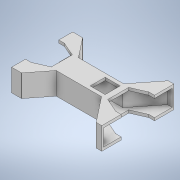
# Autodesk Inventor part: Metal_Shroud
Saved by Autodesk Inventor 2022 (Build 260153000, 153)
## iProperties
Created: 2022-01-23
Part Number: Metal_Shroud
Material: Generic
Document SubType Name: Modeling
Designer: Mlees
Density: 1 g/cm^3
Appearance: Default
Author: Mlees
Autodesk Inventor part; units mm, degrees
ref_plane "YZ Plane" through (0, 0, 0) normal (1, 0, 0) x (0, 1, 0)
ref_plane "XZ Plane" through (0, 0, 0) normal (0, 1, 0) x (-1, 0, 0)
ref_plane "XY Plane" through (0, 0, 0) normal (0, 0, 1) x (1, 0, 0)
sketch "Sketch1" plane through (0, 0, 0) normal (0, 1, 0) x (-1, 0, 0)
  line L0 (172.412, 0) -> (172.412, -65)
  line L1 (172.412, 0) -> (172.412, 65)
  line L2 (172.412, 65) -> (162.412, 65)
  line L3 (162.412, 65) -> (127.012, 20)
  line L4 (172.412, -65) -> (162.412, -65)
  line L5 (162.412, -65) -> (127.012, -20)
  line L6 (127.012, -20) -> (86.206, -20)
  line L7 (127.012, 20) -> (86.206, 20)
  line L8 (0, 0) -> (0, -65)
  line L9 (0, 0) -> (0, 65)
  line L10 (0, 65) -> (10, 65)
  line L11 (10, 65) -> (45.4, 20)
  line L12 (0, -65) -> (10, -65)
  line L13 (10, -65) -> (45.4, -20)
  line L14 (45.4, -20) -> (86.206, -20)
  line L15 (45.4, 20) -> (86.206, 20)
  dimension "d0" = 172.412
  dimension "d1" = 65
  dimension "d2" = 65
  dimension "d7" = 10
  constraints: 32 end point, 2 horizontal, 2 vertical
  measures "d0" distance of point (0, 0) L0.start
  measures "d1" distance of L0.start L0.end
  measures "d2" distance of L0.start L1.end
  measures "d7" distance of L1.end L2.end
extrude "Extrusion1" add sketch "Sketch1" along normal blind 5
sketch "Sketch2" plane through (0, 5, 0) normal (0, 1, 0) x (1, 0, 0)
  line L0 (-162.412, -65) -> (-127.012, -20) projected
  line L1 (-127.012, -20) -> (-162.412, -65)
  line L2 (-162.412, -65) -> (-172.412, -65)
  line L3 (-127.012, 20) -> (-162.412, 65) projected
  line L4 (-172.412, 65) -> (-162.412, 65)
  line L5 (-162.412, 65) -> (-127.012, 20)
  line L6 (-127.012, 20) -> (-45.4, 20)
  line L7 (-10, 65) -> (-45.4, 20) projected
  line L8 (-45.4, 20) -> (-10, 65)
  line L9 (-10, 65) -> (0, 65)
  line L10 (0, -65) -> (0, 65) projected
  line L11 (-45.4, -20) -> (-10, -65) projected
  line L12 (0, -65) -> (-10, -65)
  line L13 (-10, -65) -> (-45.4, -20)
  line L14 (-45.4, -20) -> (-127.012, -20)
  line L15 (-128.469, -17) -> (-163.869, -62)
  line L16 (-163.869, -62) -> (-169.412, -62)
  line L17 (-169.412, 62) -> (-163.869, 62)
  line L18 (-163.869, 62) -> (-128.469, 17)
  line L19 (-128.469, 17) -> (-43.943, 17)
  line L20 (-43.943, 17) -> (-8.543, 62)
  line L21 (-8.543, 62) -> (-3, 62)
  line L22 (-3, -62) -> (-8.543, -62)
  line L23 (-8.543, -62) -> (-43.943, -17)
  line L24 (-43.943, -17) -> (-128.469, -17)
  line L25 (-3, -62) -> (0, -62)
  line L26 (0, -65) -> (0, -62)
  line L27 (-3, 62) -> (0, 62)
  line L28 (0, 65) -> (0, 62)
  line L29 (-169.412, -62) -> (-172.412, -62)
  line L30 (-172.412, -65) -> (-172.412, -62)
  line L31 (-169.412, 62) -> (-172.412, 62)
  line L32 (-172.412, 62) -> (-172.412, 65)
  point P0 (0, 0)
  dimension "d10" = 3
  constraints: 56 end point, 6 parallel, 4 collinear, 3 perpendicular, 1 point on line, 1 vertical, 7 other
  measures "d10" distance between parallel lines of L14 L24
extrude "Extrusion2" add sketch "Sketch2" along normal blind 30
sketch "Sketch3" plane through (0, 35, 0) normal (0, 1, 0) x (1, 0, 0)
  line L0 (-172.412, 65) -> (-172.412, -65) projected
  line L1 (-172.412, -65) -> (-172.412, 65)
  line L2 (-162.412, 65) -> (-172.412, 65) projected
  line L3 (-172.412, 65) -> (-162.412, 65)
  line L4 (-45.4, 20) -> (-127.012, 20) projected
  line L5 (-162.412, 65) -> (-127.012, 20)
  line L6 (-127.012, 20) -> (-45.4, 20)
  line L7 (-45.4, 20) -> (-10, 65)
  line L8 (0, 65) -> (-10, 65) projected
  line L9 (-10, 65) -> (0, 65)
  line L10 (-10, -65) -> (0, -65) projected
  line L11 (0, 65) -> (0, -65)
  line L12 (0, -65) -> (-10, -65)
  line L13 (-127.012, -20) -> (-45.4, -20) projected
  line L14 (-10, -65) -> (-45.4, -20)
  line L15 (-45.4, -20) -> (-127.012, -20)
  line L16 (-162.412, -65) -> (-127.012, -20) projected
  line L17 (-127.012, -20) -> (-162.412, -65)
  line L18 (-172.412, -65) -> (-162.412, -65) projected
  line L19 (-162.412, -65) -> (-172.412, -65)
  point P0 (0, 0)
  constraints: 24 end point, 6 collinear, 2 parallel, 1 perpendicular, 1 vertical
extrude "Extrusion3" add sketch "Sketch3" along normal blind 5
sketch "Sketch4" plane through (0, 40, 0) normal (0, 1, 0) x (1, 0, 0)
  line L0 (0, 0) -> (0, -30)
  line L1 (0, -62) -> (0, 62) projected
  line L2 (0, 0) -> (0, 30)
  line L3 (0, 30) -> (-10, 30)
  line L4 (-35.4, 0) -> (-35.4, 18.85)
  line L5 (-35.4, 18.85) -> (-10, 30)
  line L6 (-35.4, 0) -> (-35.4, -18.85)
  line L7 (-35.4, -18.85) -> (-10, -30)
  line L8 (-10, -30) -> (0, -30)
  line L9 (-127.012, -20) -> (-45.4, -20) projected
  line L10 (-45.4, 20) -> (-127.012, 20) projected
  line L11 (-172.412, 0) -> (-172.412, -30)
  line L12 (-172.412, 0) -> (-172.412, 30)
  line L13 (-172.412, 30) -> (-162.412, 30)
  line L14 (-137.012, 0) -> (-137.012, 18.85)
  line L15 (-137.012, 18.85) -> (-162.412, 30)
  line L16 (-137.012, 0) -> (-137.012, -18.85)
  line L17 (-137.012, -18.85) -> (-162.412, -30)
  line L18 (-162.412, -30) -> (-172.412, -30)
  dimension "d15" = 30
  dimension "d16" = 30
  dimension "d17" = 10
  dimension "d18" = 35.4
  dimension "d19" = 18.85
  dimension "d20" = 18.85
  constraints: 32 end point, 2 perpendicular, 2 point on line, 2 vertical
  measures "d15" distance of L0.start L0.end
  measures "d16" distance of L0.start L2.end
  measures "d17" distance of L2.end L3.end
  measures "d18" distance of L0.start L4.start
  measures "d19" distance of L4.start L4.end
  measures "d20" distance of L4.start L6.end
extrude "Extrusion4" cut sketch "Sketch4" against normal through all
sketch "Sketch5" plane through (0, 40, 0) normal (0, 1, 0) x (1, 0, 0)
  line L0 (-172.412, -65) -> (-162.412, -65) projected
  line L1 (-172.412, -65) -> (-172.412, -55)
  line L2 (-172.412, -30) -> (-172.412, -65) projected
  line L3 (-162.412, 65) -> (-172.412, 65) projected
  line L4 (-172.412, 65) -> (-172.412, 55)
  line L5 (-172.412, 65) -> (-172.412, 30) projected
  line L6 (-172.412, 55) -> (-154.5453, 55)
  line L7 (-127.012, 20) -> (-162.412, 65) projected
  line L8 (-172.412, -55) -> (-154.5453, -55)
  line L9 (-162.412, -65) -> (-127.012, -20) projected
  point P0 (0, 0)
  dimension "d23" = 10
  dimension "d24" = 10
  constraints: 8 end point, 4 point on line, 1 parallel, 1 perpendicular
  measures "d23" distance of L0.start L1.end
  measures "d24" distance of L3.end L4.end
extrude "Extrusion5" cut sketch "Sketch5" against normal through all
sketch "Sketch6" plane through (-172.412, 35, 30) normal (-1, 0, 0) x (0, 0, 1)
  line L0 (-85, 5) -> (-60, 5) projected
  line L1 (-50, -35) -> (-85, -35) projected
  line L2 (-85, 5) -> (-82, 5)
  line L3 (-82, 5) -> (-82, -35)
  line L4 (-82, -35) -> (-85, -35)
  line L5 (-85, -35) -> (-85, 5)
  line L6 (25, -35) -> (-10, -35) projected
  line L7 (25, 5) -> (22, 5)
  line L8 (22, 5) -> (22, -35)
  line L9 (22, -35) -> (25, -35)
  line L10 (25, -35) -> (25, 5)
  point P0 (-30, -35)
  dimension "d27" = 3
  dimension "d28" = 3
  constraints: 16 end point, 4 parallel, 2 horizontal, 2 perpendicular, 2 point on line
  measures "d27" distance of L3.end L4.end
  measures "d28" distance of L9.end L8.end
extrude "Extrusion6" add sketch "Sketch6" against normal blind 18
sketch "Sketch7" plane through (0, 40, 0) normal (0, 1, 0) x (1, 0, 0)
  line L0 (-35.4, 18.85) -> (-35.4, -18.85) projected
  line L1 (-45.4, 13.5) -> (-72.4, 13.5)
  line L2 (-72.4, 13.5) -> (-72.4, -13.5)
  line L3 (-72.4, -13.5) -> (-45.4, -13.5)
  line L4 (-45.4, -13.5) -> (-45.4, 13.5)
  point P0 (0, 0)
  dimension "d33" = 27
  dimension "d34" = 27
  constraints: 8 end point, 2 parallel, 1 horizontal, 1 perpendicular
  measures "d33" distance of L3.end L2.end
  measures "d34" distance of L2.end L1.end
extrude "Extrusion7" cut sketch "Sketch7" against normal blind 18
body "Solid1"
